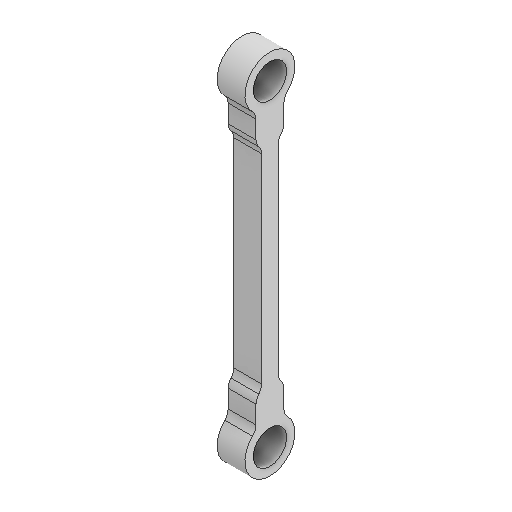
# Autodesk Inventor part: Link_DE
Saved by Autodesk Inventor 2026.2 (Build 302298000, 298)
## iProperties
Created: 2025-12-27
Part Number: Link_DE
Material: 一般
Document SubType Name: Modeling
Designer: Hsiangyu
Density: 1 g/cm^3
Appearance: 預設
Author: Hsiangyu
Autodesk Inventor part; units mm, degrees
ref_plane "YZ Plane" through (0, 0, 0) normal (1, 0, 0) x (0, 1, 0)
ref_plane "XZ Plane" through (0, 0, 0) normal (0, 1, 0) x (-1, 0, 0)
ref_plane "XY Plane" through (0, 0, 0) normal (0, 0, 1) x (1, 0, 0)
sketch "草圖1" plane through (0, 0, 0) normal (1, 0, 0) x (0, 1, 0)
  line L0 (0, 0) -> (113.9, 0)
  circle A0 centre (113.9, 0) radius 6
  circle A1 centre (0, 0) radius 6
  circle A2 centre (0, 0) radius 9
  circle A3 centre (113.9, 0) radius 9
  line L1 (7.4833, 5) -> (17.4833, 5)
  line L2 (17.4833, 5) -> (19.4833, 3)
  line L3 (19.4833, 3) -> (94.4167, 3)
  line L4 (94.4167, 3) -> (96.4167, 5)
  line L5 (96.4167, 5) -> (106.4167, 5)
  line L6 (106.4167, -5) -> (96.4167, -5)
  line L7 (96.4167, -5) -> (94.4167, -3)
  line L8 (94.4167, -3) -> (19.4833, -3)
  line L9 (19.4833, -3) -> (17.4833, -5)
  line L10 (17.4833, -5) -> (7.4833, -5)
  dimension "d0" = 113.9
  dimension "d1" = 12
  dimension "d2" = 12
  dimension "d3" = 18
  dimension "d4" = 18
  dimension "d5" = 3
  dimension "d6" = 5
  dimension "d7" = 10
  dimension "d8" = 10
  constraints: 22 end point, 6 vertical alignment, 4 centre point, 4 coincident, 4 point on circle, 4 point on line, 3 parallel, 3 perpendicular, 2 horizontal
  measures "d0" distance of L0.start L0.end
  measures "d1" diameter of A0
  measures "d2" diameter of A1
  measures "d3" diameter of A2
  measures "d4" diameter of A3
  measures "d5" distance between parallel lines of L0 L8
  measures "d6" distance between parallel lines of L0 L6
  measures "d7" distance of L6.start L6.end
  measures "d8" distance of L9.end L10.end
extrude "擠出1" add sketch "草圖1" along normal blind 10
fillet "圓角1" radius 4 12 edges at (5, 106.4167, 5) (5, 96.4167, 5) (5, 94.4167, 3) (5, 17.4833, 5) (5, 7.4833, 5) (5, 19.4833, 3) (5, 7.4833, -5) (5, 17.4833, -5) (5, 19.4833, -3) (5, 106.4167, -5) (5, 96.4167, -5) (5, 94.4167, -3)
equation "\"d2\" = d1"
equation "\"d3\" = d4"
equation "\"d8\" = d7"
